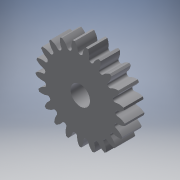
# Autodesk Inventor part: SmallGear
Saved by Autodesk Inventor 2019 (Build 230136000, 136)
## iProperties
Created: 2019-05-16
Part Number: SmallGear
Material: Generic
Document SubType Name: Modeling
Designer: Henry
Density: 1 g/cm^3
Appearance: Default
Author: Henry
Autodesk Inventor part; units mm, degrees
ref_plane "YZ Plane" through (0, 0, 0) normal (1, 0, 0) x (0, 1, 0)
ref_plane "XZ Plane" through (0, 0, 0) normal (0, 1, 0) x (-1, 0, 0)
ref_plane "XY Plane" through (0, 0, 0) normal (0, 0, 1) x (1, 0, 0)
sketch "Sketch1" plane through (0, 0, 0) normal (0, 0, 1) x (1, 0, 0)
  spline S0 degree 3 poles (-0.574, 4.5611) (-0.5592, 4.5419) (-0.5297, 4.5035) (-0.4878, 4.444) (-0.4478, 4.3833) (-0.4102, 4.321) (-0.3751, 4.2573) (-0.3429, 4.1921) (-0.3139, 4.1254) (-0.293, 4.0685) (-0.2788, 4.0222) (-0.2698, 3.9869) (-0.2623, 3.9513) (-0.26, 3.915) (-0.2547, 3.879) (-0.2482, 3.8432) (-0.2382, 3.8082) (-0.2261, 3.7739) (-0.2102, 3.7411) (-0.1907, 3.7104) (-0.1706, 3.6876) (-0.1529, 3.671) (-0.1336, 3.6563) (-0.1072, 3.641) (-0.0784, 3.6312) (-0.0545, 3.627) (-0.0303, 3.6251) (0, 3.6262) (0.0303, 3.6251) (0.0545, 3.627) (0.0784, 3.6312) (0.1072, 3.641) (0.1336, 3.6563) (0.1529, 3.671) (0.1706, 3.6876) (0.1907, 3.7104) (0.2102, 3.7411) (0.2261, 3.7739) (0.2382, 3.8082) (0.2482, 3.8432) (0.2547, 3.879) (0.26, 3.915) (0.2623, 3.9513) (0.2698, 3.9869) (0.2788, 4.0222) (0.293, 4.0685) (0.3139, 4.1254) (0.3429, 4.1921) (0.3751, 4.2573) (0.4102, 4.321) (0.4478, 4.3833) (0.4878, 4.444) (0.5297, 4.5035) (0.5592, 4.5419) (0.574, 4.5611) knots 0 0 0 0 0.031255 0.062511 0.093767 0.125022 0.156277 0.187531 0.218785 0.250036 0.265664 0.281291 0.296916 0.312542 0.328169 0.343795 0.359419 0.375041 0.390665 0.406285 0.421898 0.429707 0.437523 0.453136 0.468748 0.476563 0.484371 0.5 0.515629 0.523437 0.531252 0.546864 0.562477 0.570293 0.578102 0.593715 0.609335 0.624959 0.640581 0.656205 0.671831 0.687458 0.703084 0.718709 0.734336 0.749964 0.781215 0.812469 0.843723 0.874978 0.906233 0.937489 0.968745 1 1 1 1
  circle A0 centre (0, 0) radius 3.6257 construction
  circle A1 centre (0, 0) radius 3.9467 construction
  circle A2 centre (0, 0) radius 4.2 construction
  circle A3 centre (0, 0) radius 4.5971
  point P0 (-0.5301, 4.5032)
  point P1 (-0.4881, 4.4438)
  point P2 (-0.4482, 4.383)
  point P3 (-0.4106, 4.3208)
  point P4 (-0.3756, 4.2571)
  point P5 (-0.3434, 4.1919)
  point P6 (-0.3145, 4.1252)
  point P7 (-0.2897, 4.0569)
  point P8 (-0.2791, 4.0221)
  point P9 (-0.2701, 3.9869)
  point P10 (-0.2632, 3.9512)
  point P11 (-0.2595, 3.915)
  point P12 (-0.2545, 3.879)
  point P13 (-0.2476, 3.8433)
  point P14 (-0.2379, 3.8083)
  point P15 (-0.2255, 3.7742)
  point P16 (-0.2096, 3.7414)
  point P17 (-0.1899, 3.7109)
  point P18 (-0.166, 3.6836)
  point P19 (-0.1527, 3.6712)
  point P20 (-0.1383, 3.6601)
  point P21 (-0.1067, 3.6421)
  point P22 (-0.0724, 3.6304)
  point P23 (-0.0545, 3.6273)
  point P24 (-0.0364, 3.6258)
  point P25 (0, 3.6257)
  point P26 (0.0364, 3.6258)
  point P27 (0.0545, 3.6273)
  point P28 (0.0724, 3.6304)
  point P29 (0.1067, 3.6421)
  point P30 (0.1383, 3.6601)
  point P31 (0.1527, 3.6712)
  point P32 (0.166, 3.6836)
  point P33 (0.1899, 3.7109)
  point P34 (0.2096, 3.7414)
  point P35 (0.2255, 3.7742)
  point P36 (0.2379, 3.8083)
  point P37 (0.2476, 3.8433)
  point P38 (0.2545, 3.879)
  point P39 (0.2595, 3.915)
  point P40 (0.2632, 3.9512)
  point P41 (0.2701, 3.9869)
  point P42 (0.2791, 4.0221)
  point P43 (0.2897, 4.0569)
  point P44 (0.3145, 4.1252)
  point P45 (0.3434, 4.1919)
  point P46 (0.3756, 4.2571)
  point P47 (0.4106, 4.3208)
  point P48 (0.4482, 4.383)
  point P49 (0.4881, 4.4438)
  point P50 (0.5301, 4.5032)
  constraints: 4 centre point, 2 point on circle, 111 other
extrude "Extrusion1" add sketch "Sketch1" against normal blind 2
extrude "Extrusion2" cut sketch "Sketch1" against normal blind 2 contours A3 S0 picked at (-0.0851, 4.3061)
pattern_circular "Circular Pattern1" count 21 over 360 about axis through (0, 0, 0) along (0, 0, -1) of "Extrusion2"
sketch "Sketch2" plane through (0, 0, 0) normal (0, 0, 1) x (1, 0, 0)
  point P0 (0, 0)
sketch "Sketch3" plane through (0, 0, 0) normal (0, 0, 1) x (1, 0, 0)
  circle A0 centre (0, 0) radius 1
  dimension "d7" = 2
  constraints: 1 centre point, 1 coincident
  measures "d7" diameter of A0
extrude "Extrusion3" cut sketch "Sketch3" against normal blind 2
equation "\"d0\" = FaceWidth"
equation "\"Module\" = 0.4"
equation "\"PressureAngle\" = 20deg"
equation "\"UnitProfileClearance\" = 0.25"
equation "\"UnitRoundRadius\" = 0.35"
equation "\"HeadDiameter\" = 9.19417"
equation "\"RootDiameter\" = 7.25147"
equation "\"BaseDiameter\" = 7.89342"
equation "\"PitchDiameter\" = 8.4"
equation "\"FaceWidth\" = 2"
equation "\"HelixAngle\" = 0"
equation "\"UnitCorrection\" = 0"
equation "\"UnitAddendumModification\" = 0.007289"
equation "\"CircularPitch\" = 1.25664"
equation "\"UnitBacklashShift\" = -0.185662"
equation "\"TotalToolShift\" = -0.07426"
equation "\"IsInternal\" = 0"
body "Solid1"
